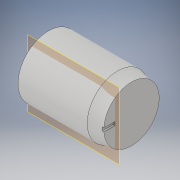
# Autodesk Inventor part: Practica 2
Saved by Autodesk Inventor 2019.1 (Build 231200000, 200)
## iProperties
Created: 2024-02-06
Part Number: Practica 2
Material: Generic
Document SubType Name: Modeling
Designer: clariheelen
Density: 1 g/cm^3
Appearance: Default
Author: clariheelen
Autodesk Inventor part; units mm, degrees
ref_plane "YZ Plane" through (0, 0, 0) normal (1, 0, 0) x (0, 1, 0)
ref_plane "XZ Plane" through (0, 0, 0) normal (0, 1, 0) x (-1, 0, 0)
sketch "Sketch2" plane through (0, 0, 0) normal (0, 0, 1) x (1, 0, 0)
  line L0 (0, 0) -> (0, 200)
  arc A0 (-100, 220) -> (0, 200) centre (-6.2023, 428.9887) ccw
  line L1 (-100, 220) -> (-600, 220)
  line L2 (-600, 220) -> (-600, 0)
  line L3 (-600, 0) -> (0, 0)
  dimension "d4" = 200
  dimension "d7" = 500
  constraints: 8 end point, 2 perpendicular, 2 point on circle, 1 centre point, 1 horizontal, 1 vertical
  measures "d4" distance of L0.start L0.end
  measures "d7" distance of L1.start L1.end
revolve "Revolution1" add sketch "Sketch2" angle 360 about axis through (-600, 0, 0) along (1, 0, 0)
ref_plane "Work Plane1" through (0, 0, 120) normal (0, 0, 1) x (1, 0, 0)
sketch "Sketch3" plane through (0, 0, 120) normal (0, 0, 1) x (1, 0, 0)
  line L0 (12.5, -12.5) -> (-12.5, -12.5)
  line L1 (-12.5, -12.5) -> (-12.5, 12.5)
  line L2 (-12.5, 12.5) -> (12.5, 12.5)
  line L3 (12.5, 12.5) -> (12.5, -12.5)
  line L4 (12.5, -12.5) -> (-12.5, 12.5) construction
  line L5 (-12.5, -12.5) -> (12.5, 12.5) construction
  point P0 (0, 0)
  dimension "d10" = 25
  dimension "d11" = 25
  constraints: 12 end point, 2 midpoint, 2 parallel, 1 horizontal, 1 perpendicular
  measures "d10" distance of L1.end L2.end
  measures "d11" distance of L0.end L1.end
extrude "Extrusion1" cut sketch "Sketch3" along normal blind 200
body "Solid1"
